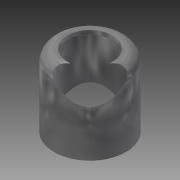
# Autodesk Inventor part: anode-bell
Saved by Autodesk Inventor 2015 (Build 190159000, 159)
## iProperties
Created: 2014-09-24
Part Number: anode-bell
Material: Stainless Steel
Document SubType Name: Modeling
Designer: Adam
Density: 8 g/cm^3
Appearance: Semi-Polished
Author: Adam
Autodesk Inventor part; units mm, degrees
ref_plane "YZ Plane" through (0, 0, 0) normal (1, 0, 0) x (0, 1, 0)
ref_plane "XZ Plane" through (0, 0, 0) normal (0, 1, 0) x (-1, 0, 0)
ref_plane "XY Plane" through (0, 0, 0) normal (0, 0, 1) x (1, 0, 0)
sketch "Sketch1" plane through (0, 0, 0) normal (0, 0, 1) x (1, 0, 0)
  line L0 (11.5, 9) -> (11.5, 6) construction
  arc A0 (11.5, 6) -> (13.5, 6) centre (12.5, 6) ccw construction
  line L1 (13.5, 6) -> (13.5, 19.8063) construction
  arc A1 (13.5, 19.8063) -> (12, 21.3063) centre (12, 19.8063) ccw construction
  arc A2 (12, 24.3063) -> (12, 21.3063) centre (12, 22.8063) ccw construction
  arc A3 (12, 24.3063) -> (13.5, 25.8063) centre (12, 25.8063) ccw construction
  line L2 (13.5, 25.8063) -> (13.5, 71) construction
  arc A4 (13.5, 71) -> (11.5, 73) centre (11.5, 71) ccw construction
  line L3 (11.5, 73) -> (2, 73) construction
  line L4 (2, 73) -> (2, 80) construction
  arc A5 (2, 80) -> (1.2, 81.6) centre (0, 80) ccw construction
  arc A6 (0, 84) -> (1.2, 81.6) centre (3, 84) ccw construction
  arc A7 (-1.2, 81.6) -> (0, 84) centre (-3, 84) ccw construction
  arc A8 (-1.2, 81.6) -> (-2, 80) centre (0, 80) ccw construction
  line L5 (-2, 80) -> (-2, 73) construction
  line L6 (-2, 73) -> (-11.5, 73) construction
  arc A9 (-11.5, 73) -> (-13.5, 71) centre (-11.5, 71) ccw construction
  line L7 (-13.5, 71) -> (-13.5, 25.8063) construction
  arc A10 (-13.5, 25.8063) -> (-12, 24.3063) centre (-12, 25.8063) ccw construction
  arc A11 (-12, 21.3063) -> (-12, 24.3063) centre (-12, 22.8063) ccw construction
  arc A12 (-12, 21.3063) -> (-13.5, 19.8063) centre (-12, 19.8063) ccw construction
  line L8 (-13.5, 19.8063) -> (-13.5, 6) construction
  arc A13 (-13.5, 6) -> (-11.5, 6) centre (-12.5, 6) ccw construction
  line L9 (-11.5, 6) -> (-11.5, 9) construction
  arc A14 (-9.5, 11) -> (-11.5, 9) centre (-9.5, 9) ccw construction
  line L10 (-9.5, 11) -> (-9.5, 6) construction
  arc A15 (-15.5, 6) -> (-9.5, 6) centre (-12.5, 6) ccw construction
  line L11 (-15.5, 6) -> (-15.5, 19.8063) construction
  arc A16 (-13.8028, 22.8063) -> (-15.5, 19.8063) centre (-12, 19.8063) ccw construction
  arc A17 (-15.5, 25.8063) -> (-13.8028, 22.8063) centre (-12, 25.8063) ccw construction
  line L12 (-15.5, 25.8063) -> (-15.5, 71) construction
  arc A18 (-11.5, 75) -> (-15.5, 71) centre (-11.5, 71) ccw construction
  line L13 (-11.5, 75) -> (-3, 75) construction
  line L14 (-3, 75) -> (-3, 80) construction
  arc A19 (-1.8, 82.4) -> (-3, 80) centre (0, 80) ccw construction
  arc A20 (-1.8, 82.4) -> (-1, 84) centre (-3, 84) ccw construction
  arc A21 (0, 85) -> (-1, 84) centre (0, 84) ccw construction
  arc A22 (1, 84) -> (0, 85) centre (0, 84) ccw construction
  arc A23 (1, 84) -> (1.8, 82.4) centre (3, 84) ccw construction
  arc A24 (3, 80) -> (1.8, 82.4) centre (0, 80) ccw construction
  line L15 (3, 80) -> (3, 75) construction
  line L16 (3, 75) -> (11.5, 75) construction
  arc A25 (15.5, 71) -> (11.5, 75) centre (11.5, 71) ccw construction
  line L17 (15.5, 71) -> (15.5, 25.8063) construction
  arc A26 (13.8028, 22.8063) -> (15.5, 25.8063) centre (12, 25.8063) ccw construction
  arc A27 (15.5, 19.8063) -> (13.8028, 22.8063) centre (12, 19.8063) ccw construction
  line L18 (15.5, 19.8063) -> (15.5, 6) construction
  arc A28 (9.5, 6) -> (15.5, 6) centre (12.5, 6) ccw construction
  line L19 (9.5, 6) -> (9.5, 11) construction
  arc A29 (11.5, 9) -> (9.5, 11) centre (9.5, 9) ccw construction
  line L20 (-9.5, 6) -> (-8.5, 6)
  line L21 (-8.5, 6) -> (-8.5, 22)
  line L22 (-9.5, 22) -> (-9.5, 6)
  arc A30 (-6.5, 25) -> (-9.5, 22) centre (-6.5, 22) ccw
  arc A31 (-6.5, 24) -> (-8.5, 22) centre (-6.5, 22) ccw
  line L23 (-6, 25) -> (-6.5, 25)
  line L24 (-6, 24) -> (-6.5, 24)
  line L25 (5.1354, 22) -> (-7.1821, 22) construction
  line L26 (0, 22) -> (0, 0) construction
  line L27 (-6, 25) -> (-6, 24)
  dimension "d0" = 1
  dimension "d2" = 18
  dimension "d3" = 6
  dimension "d4" = 2
  dimension "d5" = 6
  constraints: 64 point on circle, 56 end point, 32 centre point, 17 vertical, 6 horizontal, 4 tangent, 3 point on line, 2 parallel, 2 perpendicular, 1 coincident, 110 other
  measures "d0" distance between parallel lines of L22 L21
  measures "d2" distance between parallel lines of L20 L24
  measures "d3" distance from line of L26.end L20
  measures "d4" radius of A31
  measures "d5" distance between parallel lines of L26 L27
revolve "Revolution1" add sketch "Sketch1" angle 360 about axis through (0, 22, 0) along (0, -1, 0)
equation "\"d0\" = d1"
equation "\"d1\" = 1"
body "Solid1"
